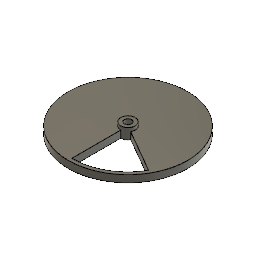
cap (Autodesk Fusion 360 design; units mm, degrees)
Autodesk Fusion 360 part; units mm, degrees
sketch "Sketch3" plane through (0, 0, 0) normal (0, 1, 0) x (1, 0, 0)
  circle A0 centre (0, 0) radius 33
  circle A1 centre (0, 0) radius 31
  line L0 (0, 0) -> (0, -31)
  line L1 (0, 0) -> (26.8468, -15.5)
  line L2 (0, 0) -> (31, 0) construction
  circle A2 centre (0, 0) radius 4
  dimension "d8" = 66
  dimension "d9" = 62
  dimension "d10" = 30
  dimension "d11" = 8
  measures "d8" diameter of A0
  measures "d9" diameter of A1
  measures "d10" angle of L1 L2
  measures "d11" diameter of A2
extrude "Extrude3" add sketch "Sketch3" along normal blind 4 contours A0 | A1 L0 L1 A2 | L0 L1 A2 | L0 L1 A2 picked at (-10.729, -19.1384)
sketch "Sketch4" plane through (0, 4, 0) normal (0, 1, 0) x (-1, 0, 0)
  arc A0 (0, 31) -> (-26.8468, 15.5) centre (0, 0) ccw
  line L0 (0, 31) -> (0, 4)
  arc A1 (0, 4) -> (-3.4641, 2) centre (0, 0) ccw
  line L1 (-3.4641, 2) -> (-26.8468, 15.5)
  circle A2 centre (0, 0) radius 33
  circle A3 centre (0, 0) radius 2
  circle A4 centre (0, 0) radius 4
  dimension "d14" = 4
  dimension "d15" = 8
  measures "d14" diameter of A3
  measures "d15" diameter of A4
extrude "Extrude4" add sketch "Sketch4" along normal blind 2 contours A1 A4
extrude "Extrude5" cut 1 faces at (-0.2436, 4, -0.2863) along direction (0, -1, 0) blind 2
